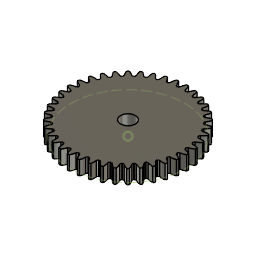
Second gear (Autodesk Fusion 360 design; units mm, degrees)
part number: 2026-05-11-16-26-52-413
Autodesk Fusion 360 part; units mm, degrees
sketch "Base Circle" plane through (0, 0, 0) normal (0, 0, 1) x (1, 0, 0)
  circle A0 centre (0, 0) radius 18.843
  circle A1 centre (0, 0) radius 2.6
extrude "Extrude3" add sketch "Base Circle" along normal blind 5
sketch "Gear Tooth" plane through (0, 0, 0) normal (0, 0, 1) x (1, 0, 0)
  spline S0 degree 5 poles (18.7675, -0.9942) (18.7739, -0.9942) (18.7867, -0.9943) (18.806, -0.9942) (18.8316, -0.9937) (18.8636, -0.9926) (18.8957, -0.991) (18.9278, -0.9888) (18.9598, -0.9862) (18.9919, -0.9831) (19.024, -0.9796) (19.0561, -0.9758) (19.0882, -0.9716) (19.1203, -0.9672) (19.1524, -0.9625) (19.1845, -0.9575) (19.2166, -0.9522) (19.2487, -0.9467) (19.2808, -0.941) (19.3129, -0.935) (19.345, -0.9287) (19.377, -0.9222) (19.4091, -0.9155) (19.4412, -0.9086) (19.4732, -0.9014) (19.5053, -0.8941) (19.5373, -0.8865) (19.5693, -0.8787) (19.6014, -0.8708) (19.6334, -0.8626) (19.6654, -0.8542) (19.6974, -0.8457) (19.7294, -0.8369) (19.7613, -0.828) (19.7933, -0.8189) (19.8252, -0.8096) (19.8572, -0.8001) (19.8891, -0.7905) (19.921, -0.7806) (19.9529, -0.7707) (19.9848, -0.7605) (20.0167, -0.7502) (20.0486, -0.7397) (20.0804, -0.729) (20.1123, -0.7182) (20.1441, -0.7072) (20.1759, -0.696) (20.2077, -0.6847) (20.2395, -0.6733) (20.2712, -0.6617) (20.303, -0.6499) (20.3347, -0.638) (20.3664, -0.6259) (20.3981, -0.6137) (20.4298, -0.6013) (20.4615, -0.5888) (20.4932, -0.5761) (20.5248, -0.5633) (20.5564, -0.5503) (20.588, -0.5372) (20.6196, -0.5239) (20.6511, -0.5106) (20.6827, -0.497) (20.7142, -0.4833) (20.7457, -0.4695) (20.7772, -0.4556) (20.8087, -0.4415) (20.8401, -0.4273) (20.8715, -0.4129) (20.9029, -0.3984) (20.9343, -0.3838) (20.9594, -0.372) (20.9782, -0.363) (20.9907, -0.3571) (20.997, -0.3541) knots 0 0 0 0 0 0 0.01428571 0.02857143 0.04285714 0.05714286 0.07142857 0.08571429 0.1 0.11428571 0.12857143 0.14285714 0.15714286 0.17142857 0.18571429 0.2 0.21428571 0.22857143 0.24285714 0.25714286 0.27142857 0.28571429 0.3 0.31428571 0.32857143 0.34285714 0.35714286 0.37142857 0.38571429 0.4 0.41428571 0.42857143 0.44285714 0.45714286 0.47142857 0.48571429 0.5 0.51428571 0.52857143 0.54285714 0.55714286 0.57142857 0.58571429 0.6 0.61428571 0.62857143 0.64285714 0.65714286 0.67142857 0.68571429 0.7 0.71428571 0.72857143 0.74285714 0.75714286 0.77142857 0.78571429 0.8 0.81428571 0.82857143 0.84285714 0.85714286 0.87142857 0.88571429 0.9 0.91428571 0.92857143 0.94285714 0.95714286 0.97142857 0.98571429 1 1 1 1 1 1
  spline S1 degree 5 poles (18.7675, 0.9942) (18.7739, 0.9942) (18.7867, 0.9943) (18.806, 0.9942) (18.8316, 0.9937) (18.8636, 0.9926) (18.8957, 0.991) (18.9278, 0.9888) (18.9598, 0.9862) (18.9919, 0.9831) (19.024, 0.9796) (19.0561, 0.9758) (19.0882, 0.9716) (19.1203, 0.9672) (19.1524, 0.9625) (19.1845, 0.9575) (19.2166, 0.9522) (19.2487, 0.9467) (19.2808, 0.941) (19.3129, 0.935) (19.345, 0.9287) (19.377, 0.9222) (19.4091, 0.9155) (19.4412, 0.9086) (19.4732, 0.9014) (19.5053, 0.8941) (19.5373, 0.8865) (19.5693, 0.8787) (19.6014, 0.8708) (19.6334, 0.8626) (19.6654, 0.8542) (19.6974, 0.8457) (19.7294, 0.8369) (19.7613, 0.828) (19.7933, 0.8189) (19.8252, 0.8096) (19.8572, 0.8001) (19.8891, 0.7905) (19.921, 0.7806) (19.9529, 0.7707) (19.9848, 0.7605) (20.0167, 0.7502) (20.0486, 0.7397) (20.0804, 0.729) (20.1123, 0.7182) (20.1441, 0.7072) (20.1759, 0.696) (20.2077, 0.6847) (20.2395, 0.6733) (20.2712, 0.6617) (20.303, 0.6499) (20.3347, 0.638) (20.3664, 0.6259) (20.3981, 0.6137) (20.4298, 0.6013) (20.4615, 0.5888) (20.4932, 0.5761) (20.5248, 0.5633) (20.5564, 0.5503) (20.588, 0.5372) (20.6196, 0.5239) (20.6511, 0.5106) (20.6827, 0.497) (20.7142, 0.4833) (20.7457, 0.4695) (20.7772, 0.4556) (20.8087, 0.4415) (20.8401, 0.4273) (20.8715, 0.4129) (20.9029, 0.3984) (20.9343, 0.3838) (20.9594, 0.372) (20.9782, 0.363) (20.9907, 0.3571) (20.997, 0.3541) knots 0 0 0 0 0 0 0.01428571 0.02857143 0.04285714 0.05714286 0.07142857 0.08571429 0.1 0.11428571 0.12857143 0.14285714 0.15714286 0.17142857 0.18571429 0.2 0.21428571 0.22857143 0.24285714 0.25714286 0.27142857 0.28571429 0.3 0.31428571 0.32857143 0.34285714 0.35714286 0.37142857 0.38571429 0.4 0.41428571 0.42857143 0.44285714 0.45714286 0.47142857 0.48571429 0.5 0.51428571 0.52857143 0.54285714 0.55714286 0.57142857 0.58571429 0.6 0.61428571 0.62857143 0.64285714 0.65714286 0.67142857 0.68571429 0.7 0.71428571 0.72857143 0.74285714 0.75714286 0.77142857 0.78571429 0.8 0.81428571 0.82857143 0.84285714 0.85714286 0.87142857 0.88571429 0.9 0.91428571 0.92857143 0.94285714 0.95714286 0.97142857 0.98571429 1 1 1 1 1 1
  arc A0 (20.997, -0.3541) -> (20.997, 0.3541) centre (0, 0) ccw
  line L0 (18.7675, 0.9942) -> (18.7675, -0.9942)
  point P0 (18.9256, -0.9889)
  point P1 (19.0843, -0.9721)
  point P2 (19.2433, -0.9476)
  point P3 (19.4025, -0.9168)
  point P4 (19.562, -0.8805)
  point P5 (19.7215, -0.839)
  point P6 (19.8811, -0.7929)
  point P7 (20.0408, -0.7422)
  point P8 (20.2004, -0.6873)
  point P9 (20.36, -0.6283)
  point P10 (20.5195, -0.5654)
  point P11 (20.6788, -0.4986)
  point P12 (20.838, -0.4282)
  point P13 (18.9256, 0.9889)
  point P14 (19.0843, 0.9721)
  point P15 (19.2433, 0.9476)
  point P16 (19.4025, 0.9168)
  point P17 (19.562, 0.8805)
  point P18 (19.7215, 0.839)
  point P19 (19.8811, 0.7929)
  point P20 (20.0408, 0.7422)
  point P21 (20.2004, 0.6873)
  point P22 (20.36, 0.6283)
  point P23 (20.5195, 0.5654)
  point P24 (20.6788, 0.4986)
  point P25 (20.838, 0.4282)
extrude "Extrude4" add sketch "Gear Tooth" along normal blind 5
fillet "Fillet2" radius 0.5 2 edges at (18.8168, 0.9939, 2.5) (18.8168, -0.9939, 2.5)
pattern_circular "C-Pattern2" count 40 over 360 about axis through (0, 0, 0) along (0, 0, 1) of "Extrude4", "Fillet2"
sketch "Diametrial Pitch Circle" plane through (0, 0, 0) normal (0, 0, 1) x (1, 0, 0)
  circle A0 centre (0, 0) radius 20 construction
named bodies: "Spur Gear (40 teeth)"
